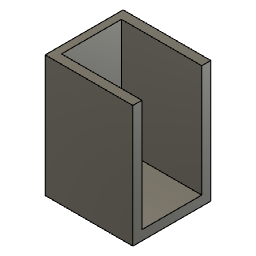
Servo Motor Hold piece v4 (Autodesk Fusion 360 design; units mm, degrees)
Autodesk Fusion 360 part; units mm, degrees
box "BoxPrimitive1" add length 25 width 16 height 18 placed x (0, 1, 0) y (0, 0, 1) z (1, 0, 0) at (0, 0, 0)
sketch "Sketch2" plane through (18, 0, 0) normal (1, 0, 0) x (0, 0, -1)
  line L0 (0, 25) -> (-16, 25)
  line L1 (-16, 25) -> (-16, 0)
  line L2 (-16, 0) -> (0, 0)
  line L3 (0, 0) -> (0, 25)
  line L4 (-8, 25) -> (-8, 13.5) construction
  line L5 (-1.85, 25) -> (-14.15, 25)
  line L6 (-14.15, 25) -> (-14.15, 2)
  line L7 (-14.15, 2) -> (-1.85, 2)
  line L8 (-1.85, 2) -> (-1.85, 25)
  line L9 (-1.85, 25) -> (-14.15, 2) construction
  line L10 (-14.15, 25) -> (-1.85, 2) construction
  point P0 (-8, 13.5)
  dimension "d12" = 11.5
  dimension "d13" = 12.3
  dimension "d14" = 23
  constraint midpoint L0 L4.start
  constraint perpendicular L0 L4
  constraint horizontal L5
  constraint perpendicular L5 L6
  constraint parallel L5 L7
  constraint parallel L6 L8
  constraint coincident L9 P0
  constraint coincident L10 P0
  constraint coincident P0 L4.end
  measures "d12" distance of L4.start P0
  measures "d13" distance of L6.end L7.end
  measures "d14" distance of L5.end L6.end
extrude "Extrude1" cut sketch "Sketch2" against normal blind 16.5 contours L0 L5 L6 L7 L8
equation "Height = 25 mm"
equation "Width = 16 mm"
equation "LengthHole = 16.5 mm"
equation "Length = 18 mm"
equation "d5 = Height"
equation "d6 = Width"
equation "d7 = Length"
equation "WidthHole = 12.3 mm"
equation "Heighthole = 23 mm"
equation "d12 = Heighthole / 2"
equation "d13 = WidthHole"
equation "d14 = Heighthole"
equation "d15 = -LengthHole"
